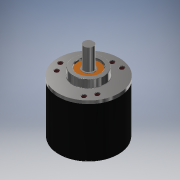
# Autodesk Inventor part: Rotary Encoder
Saved by Autodesk Inventor 2019 (Build 230136000, 136)
## iProperties
Created: 2019-06-12
Part Number: Rotary Encoder
Material: Generic
Document SubType Name: Modeling
Designer: Yuchofif
Density: 1 g/cm^3
Appearance: Default
Author: Yuchofif
Autodesk Inventor part; units mm, degrees
ref_plane "YZ Plane" through (0, 0, 0) normal (1, 0, 0) x (0, 1, 0)
ref_plane "XY Plane" through (0, 0, 0) normal (0, 0, 1) x (1, 0, 0)
sketch "Sketch1" plane through (0, 0, 0) normal (0, 0, 1) x (1, 0, 0)
  circle A0 centre (0, 0) radius 19.12
  constraints: 1 centre point, 1 coincident
extrude "Extrusion1" add sketch "Sketch1" against normal blind 34.12
fillet "Fillet1" radius 1 1 edges at (-19.12, 0, -34.12)
sketch "Sketch2" plane through (0, 0, 0) normal (0, 0, 1) x (1, 0, 0)
  circle A0 centre (0, 0) radius 19.12 projected
  circle A1 centre (0, 0) radius 19.37
  constraints: 1 centre point, 1 coincident
extrude "Extrusion2" add sketch "Sketch2" against normal blind 2
sketch "Sketch3" plane through (0, 0, 0) normal (0, 0, 1) x (1, 0, 0)
  circle A0 centre (0, 0) radius 19.37 projected
  circle A1 centre (0, 0) radius 10
  constraints: 1 centre point, 1 coincident
extrude "Extrusion3" add sketch "Sketch3" along normal blind 5 contours A1
sketch "Sketch4" plane through (0, 0, 5) normal (0, 0, 1) x (1, 0, 0)
  circle A0 centre (0, 0) radius 10 projected
  circle A1 centre (0, 0) radius 7.14
  constraints: 1 centre point, 1 coincident
extrude "Extrusion4" cut sketch "Sketch4" against normal blind 5 contours A1
sketch "Sketch5" plane through (0, 0, 0) normal (0, 0, 1) x (1, 0, 0)
  circle A0 centre (0, 0) radius 7.14 projected
  circle A1 centre (0, 0) radius 3.83
  constraints: 1 centre point, 1 coincident
extrude "Extrusion5" add sketch "Sketch5" along normal blind 4 contours A1
sketch "Sketch6" plane through (0, 0, 4) normal (0, 0, 1) x (1, 0, 0)
  circle A0 centre (0, 0) radius 3.83 projected
  circle A1 centre (0, 0) radius 3
  constraints: 1 centre point, 1 coincident
extrude "Extrusion6" add sketch "Sketch6" along normal blind 13.4 contours A1
sketch "Sketch7" plane through (0, 0, 17.4) normal (0, 0, 1) x (1, 0, 0)
  circle A0 centre (0, 0) radius 3
  line L0 (0, 2.8) -> (1.077033, 2.8)
  line L1 (0, 2.8) -> (-1.077033, 2.8)
  arc A1 (1.077033, 2.8) -> (0, 3) centre (0, 0) ccw
  arc A2 (0, 3) -> (-1.077033, 2.8) centre (0, 0) ccw
  constraints: 7 point on circle, 4 end point, 2 centre point, 2 coincident, 1 collinear
extrude "Extrusion7" cut sketch "Sketch7" against normal blind 10 contours L0 L1 A0 picked at (-0.601378, 2.836851)
fillet "Fillet2" radius 0.3 2 edges at (-10, 0, 5) (-10, 0, 0)
chamfer "Chamfer1" distance 0.3 angle 45 1 edges at (-7.14, 0, 5)
sketch "Sketch8" plane through (0, 0, 0) normal (0, 0, 1) x (1, 0, 0)
  circle A0 centre (0, 0) radius 3.83 projected
  circle A1 centre (0, 0) radius 7.14 projected
  circle A2 centre (0, 0) radius 7.1
  constraints: 1 centre point, 1 coincident
sketch "Sketch8 outline for Extrusion8" plane through (0, 0, 0) normal (0, 0, 1) x (1, 0, 0)
  circle A0 centre (0, 0) radius 7.1
  circle A1 centre (0, 0) radius 3.83
extrude "Extrusion8" add sketch "Sketch8 outline for Extrusion8" along normal blind 3.8
sketch "Sketch9" plane through (0, 0, 0) normal (0, 0, 1) x (1, 0, 0)
  circle A0 centre (0, 0) radius 19.37
  circle A1 centre (0, 14.835) radius 1.25
  circle A2 centre (-12.847487, -7.4175) radius 1.25
  circle A3 centre (12.847487, -7.4175) radius 1.25
  circle A4 centre (6.2, 14.835) radius 1.25
  circle A5 centre (-15.947487, -2.048142) radius 1.25
  circle A6 centre (9.747487, -12.786858) radius 1.25
  dimension "d32" = 360
  dimension "d38" = 360
  constraints: 6 centre point, 14 other
extrude "Extrusion9" cut sketch "Sketch9" against normal blind 5 contours A1 | A2 | A3 | A4 | A5 | A6
thread "Thread1" size "M3x0.5" class "6H" standard "ANSI Metric M Profile" full length
thread "Thread2" size "M3x0.5" class "6H" standard "ANSI Metric M Profile" full length
thread "Thread3" size "M3x0.5" class "6H" standard "ANSI Metric M Profile" full length
thread "Thread4" size "M3x0.5" class "6H" standard "ANSI Metric M Profile" full length
thread "Thread5" size "M3x0.5" class "6H" standard "ANSI Metric M Profile" full length
thread "Thread6" size "M3x0.5" class "6H" standard "ANSI Metric M Profile" full length
chamfer "Chamfer2" distance 0.3 angle 45 6 edges at (-1.25, 14.835, 0) (4.95, 14.835, 0) (11.5975, -7.4175, 0) (8.4975, -12.7869, 0) (-14.0975, -7.4175, 0) (-17.1975, -2.0481, 0)
ref_plane "Work Plane2" through (0, 21.12, 0) normal (0, 1, 0) x (-1, 0, 0)
ref_plane "Work Plane1" through (0, 19.12, 0) normal (0, 1, 0) x (-1, 0, 0)
sketch "Sketch10" plane through (0, 21.12, 0) normal (0, 1, 0) x (-1, 0, 0)
  line L0 (18.12, -34.12) -> (-18.12, -34.12) projected
  line L1 (-19.12, -33.12) -> (19.12, -33.12) projected
  line L2 (0, -33.12) -> (0, -26.12)
  circle A0 centre (0, -26.12) radius 5
  circle A1 centre (0, -26.12) radius 2.5
  point P0 (0, 0)
  constraints: 2 centre point, 2 coincident, 2 end point, 1 midpoint, 1 perpendicular
extrude "Extrusion10" add sketch "Sketch10" against normal blind 5
body "Solid1"
